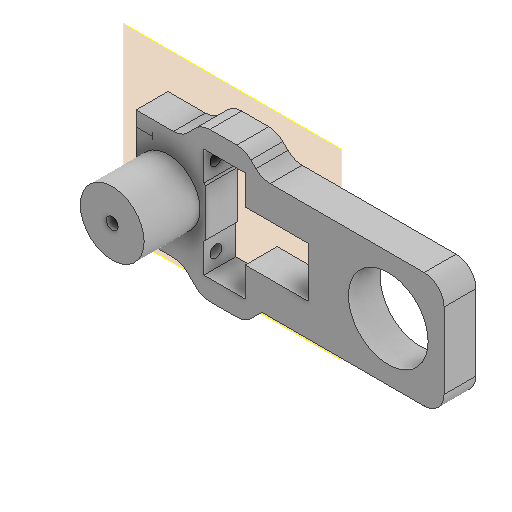
# Autodesk Inventor part: 30_Cube_Cube_Z_Focus_NEMA8_captive_objectivemount_v0
Saved by Autodesk Inventor 2022 (Build 260153000, 153)
## iProperties
Created: 2021-12-20
Part Number: 30_Cube_Cube_Z_Focus_NEMA8_captive_objectivemount_v0
Material: Generisch
Document SubType Name: Modeling
Designer: diederichbenedict
Density: 1 g/cm^3
Appearance: Vorgabe
Author: diederichbenedict
Autodesk Inventor part; units mm, degrees
ref_plane "YZ Plane" through (0, 0, 0) normal (1, 0, 0) x (0, 1, 0)
ref_plane "XZ Plane" through (0, 0, 0) normal (0, 1, 0) x (-1, 0, 0)
ref_plane "XY Plane" through (0, 0, 0) normal (0, 0, 1) x (1, 0, 0)
ref_plane "Arbeitsebene1" through (0, 0, 0) normal (0, 0, 1) x (1, 0, 0)
sketch "Skizze1" plane through (0, 0, 0) normal (0, 0, 1) x (1, 0, 0)
  arc A0 (9.5966, 13.5152) -> (9.0972, 14.0928) centre (8.4862, 13.06) ccw construction
  arc A1 (8.9755, 14.2862) -> (9.0972, 14.0928) centre (9.2245, 14.308) ccw construction
  line L0 (8.9755, 14.2862) -> (8.9453, 14.6318) construction
  arc A2 (8.9453, 14.6318) -> (8.6962, 14.86) centre (8.6962, 14.61) ccw construction
  line L1 (8.6962, 14.86) -> (8.2438, 14.86) construction
  arc A3 (8.2438, 14.86) -> (7.9947, 14.6318) centre (8.2438, 14.61) ccw construction
  line L2 (7.9947, 14.6318) -> (7.9627, 14.2652) construction
  arc A4 (7.8468, 14.0755) -> (7.9627, 14.2652) centre (7.7136, 14.287) ccw construction
  arc A5 (7.8468, 14.0755) -> (7.3759, 13.5152) centre (8.4862, 13.06) ccw construction
  arc A6 (7.1446, 13.36) -> (7.3759, 13.5152) centre (7.1446, 13.61) ccw construction
  line L3 (7.1446, 13.36) -> (6.47, 13.36) construction
  line L4 (6.47, 13.36) -> (5.97, 13.86) construction
  line L5 (5.97, 13.86) -> (5.97, 24.86) construction
  line L6 (5.97, 24.86) -> (6.47, 25.36) construction
  line L7 (6.47, 25.36) -> (7.1446, 25.36) construction
  arc A7 (7.3759, 25.2048) -> (7.1446, 25.36) centre (7.1446, 25.11) ccw construction
  arc A8 (7.3759, 25.2048) -> (7.8468, 24.6445) centre (8.4862, 25.66) ccw construction
  arc A9 (7.9627, 24.4548) -> (7.8468, 24.6445) centre (7.7136, 24.433) ccw construction
  line L8 (7.9627, 24.4548) -> (7.9947, 24.0882) construction
  arc A10 (7.9947, 24.0882) -> (8.2438, 23.86) centre (8.2438, 24.11) ccw construction
  line L9 (8.2438, 23.86) -> (8.6962, 23.86) construction
  arc A11 (8.6962, 23.86) -> (8.9453, 24.0882) centre (8.6962, 24.11) ccw construction
  line L10 (8.9453, 24.0882) -> (8.9755, 24.4338) construction
  arc A12 (9.0972, 24.6272) -> (8.9755, 24.4338) centre (9.2245, 24.412) ccw construction
  arc A13 (9.0972, 24.6272) -> (9.5966, 25.2048) centre (8.4862, 25.66) ccw construction
  arc A14 (9.8279, 25.36) -> (9.5966, 25.2048) centre (9.8279, 25.11) ccw construction
  line L11 (9.8279, 25.36) -> (10.97, 25.36) construction
  line L12 (10.97, 25.36) -> (10.97, 32.26) construction
  line L13 (10.97, 32.26) -> (10.37, 32.86) construction
  line L14 (10.37, 32.86) -> (6.97, 32.86) construction
  arc A15 (6.17, 32.86) -> (6.97, 32.86) centre (6.57, 33.16) ccw construction
  line L15 (6.17, 32.86) -> (1.57, 32.86) construction
  line L16 (1.57, 32.86) -> (0.97, 32.26) construction
  line L17 (0.97, 32.26) -> (0.97, 25.76) construction
  line L18 (0.97, 25.76) -> (1.37, 25.36) construction
  line L19 (1.37, 25.36) -> (1.37, 13.36) construction
  line L20 (1.37, 13.36) -> (0.97, 12.96) construction
  line L21 (0.97, 12.96) -> (0.97, 6.46) construction
  line L22 (0.97, 6.46) -> (1.57, 5.86) construction
  line L23 (1.57, 5.86) -> (10.37, 5.86) construction
  line L24 (10.37, 5.86) -> (10.97, 6.46) construction
  line L25 (10.97, 6.46) -> (10.97, 13.36) construction
  line L26 (10.97, 13.36) -> (9.8279, 13.36) construction
  arc A16 (9.5966, 13.5152) -> (9.8279, 13.36) centre (9.8279, 13.61) ccw construction
  line L27 (10.4528, 5.66) -> (1.4872, 5.66) construction
  line L28 (1.4872, 5.66) -> (0.77, 6.3772) construction
  line L29 (0.77, 6.3772) -> (0.77, 13.0428) construction
  line L30 (0.77, 13.0428) -> (1.17, 13.4428) construction
  line L31 (1.17, 13.4428) -> (1.17, 25.2772) construction
  line L32 (1.17, 25.2772) -> (0.77, 25.6772) construction
  line L33 (0.77, 25.6772) -> (0.77, 32.3428) construction
  line L34 (0.77, 32.3428) -> (1.4872, 33.06) construction
  line L35 (1.4872, 33.06) -> (6.2872, 33.06) construction
  arc A17 (6.2872, 33.06) -> (6.8528, 33.06) centre (6.57, 33.16) ccw construction
  line L36 (6.8528, 33.06) -> (10.4528, 33.06) construction
  line L37 (10.4528, 33.06) -> (11.17, 32.3428) construction
  line L38 (11.17, 32.3428) -> (11.17, 25.16) construction
  line L39 (11.17, 25.16) -> (9.8279, 25.16) construction
  arc A18 (9.8279, 25.16) -> (9.7816, 25.129) centre (9.8279, 25.11) ccw construction
  arc A19 (9.1991, 24.4551) -> (9.7816, 25.129) centre (8.4862, 25.66) ccw construction
  arc A20 (9.1991, 24.4551) -> (9.1747, 24.4164) centre (9.2245, 24.412) ccw construction
  line L40 (9.1747, 24.4164) -> (9.1445, 24.0708) construction
  arc A21 (8.6962, 23.66) -> (9.1445, 24.0708) centre (8.6962, 24.11) ccw construction
  line L41 (8.6962, 23.66) -> (8.2438, 23.66) construction
  arc A22 (7.7955, 24.0708) -> (8.2438, 23.66) centre (8.2438, 24.11) ccw construction
  line L42 (7.7955, 24.0708) -> (7.7634, 24.4373) construction
  arc A23 (7.7634, 24.4373) -> (7.7403, 24.4753) centre (7.7136, 24.433) ccw construction
  arc A24 (7.1909, 25.129) -> (7.7403, 24.4753) centre (8.4862, 25.66) ccw construction
  arc A25 (7.1909, 25.129) -> (7.1446, 25.16) centre (7.1446, 25.11) ccw construction
  line L43 (7.1446, 25.16) -> (6.5528, 25.16) construction
  line L44 (6.5528, 25.16) -> (6.17, 24.7772) construction
  line L45 (6.17, 24.7772) -> (6.17, 13.9428) construction
  line L46 (6.17, 13.9428) -> (6.5528, 13.56) construction
  line L47 (6.5528, 13.56) -> (7.1446, 13.56) construction
  arc A26 (7.1446, 13.56) -> (7.1909, 13.591) centre (7.1446, 13.61) ccw construction
  arc A27 (7.7403, 14.2447) -> (7.1909, 13.591) centre (8.4862, 13.06) ccw construction
  arc A28 (7.7403, 14.2447) -> (7.7634, 14.2827) centre (7.7136, 14.287) ccw construction
  line L48 (7.7634, 14.2827) -> (7.7955, 14.6492) construction
  arc A29 (8.2438, 15.06) -> (7.7955, 14.6492) centre (8.2438, 14.61) ccw construction
  line L49 (8.2438, 15.06) -> (8.6962, 15.06) construction
  arc A30 (9.1445, 14.6492) -> (8.6962, 15.06) centre (8.6962, 14.61) ccw construction
  line L50 (9.1445, 14.6492) -> (9.1747, 14.3036) construction
  arc A31 (9.1747, 14.3036) -> (9.1991, 14.2649) centre (9.2245, 14.308) ccw construction
  arc A32 (9.7816, 13.591) -> (9.1991, 14.2649) centre (8.4862, 13.06) ccw construction
  arc A33 (9.7816, 13.591) -> (9.8279, 13.56) centre (9.8279, 13.61) ccw construction
  line L51 (9.8279, 13.56) -> (11.17, 13.56) construction
  line L52 (11.17, 13.56) -> (11.17, 6.3772) construction
  line L53 (11.17, 6.3772) -> (10.4528, 5.66) construction
  line L54 (11.17, 25.66) -> (33.0091, 25.66)
  line L55 (11.17, 25.66) -> (33.0091, 25.66) construction
  line L56 (33.0091, 33.86) -> (15.3197, 33.86)
  line L57 (15.3197, 33.86) -> (11.1197, 38.06)
  line L58 (11.1197, 38.06) -> (0.1946, 38.06)
  line L59 (-16.23, 33.06) -> (-16.23, 19.36)
  line L60 (-16.23, 19.36) -> (1.17, 19.36)
  line L61 (1.17, 19.36) -> (1.17, 25.2772)
  line L62 (1.17, 25.2772) -> (0.77, 25.6772)
  line L63 (0.77, 25.6772) -> (0.77, 33.06)
  line L64 (0.77, 33.06) -> (11.17, 33.06)
  line L65 (11.17, 33.06) -> (11.17, 25.66)
  line L66 (36.7731, 34.36) -> (36.7731, 25.3561) projected
  line L67 (36.7731, 13.415) -> (36.7731, 4.36) projected
  line L68 (0.1946, 38.06) -> (-4.8054, 33.06)
  line L69 (0.1946, 38.06) -> (7.2656, 38.06) construction
  line L70 (-4.8054, 33.06) -> (-16.23, 33.06)
  line L71 (33.0091, 33.86) -> (33.0091, 25.66)
  line L72 (33.0091, 33.86) -> (61.0424, 33.86)
  line L73 (61.0424, 33.86) -> (61.0424, 19.36)
  line L74 (61.0424, 19.36) -> (57.0424, 19.36)
  line L75 (37.0424, 19.36) -> (27.0424, 19.36)
  line L76 (27.0424, 19.36) -> (27.0424, 25.66)
  circle A34 centre (47.0424, 19.36) radius 10
  point P0 (0, 0)
  point P1 (-2.0031, 19.36)
  point P2 (-4.8031, 19.36)
  dimension "d0" = 0.2
  dimension "d2" = 5
  dimension "d4" = 17
  dimension "d7" = 0.5
  dimension "d8" = 3.5
  dimension "d21" = 135
  dimension "d45" = 20
  dimension "d46" = 14
  dimension "d47" = 20
  dimension "d48" = 14.5
  constraints: 96 end point, 36 point on circle, 18 centre point, 7 point on line, 6 parallel, 4 perpendicular, 3 horizontal, 2 equal length, 1 collinear, 1 midpoint, 1 vertical, 43 other
  measures "d0" distance between parallel lines of L23 L27
  measures "d2" distance between parallel lines of L35 L58
  measures "d4" distance between parallel lines of L63 L59
  measures "d7" distance from line of L54 L38.end
  measures "d8" distance from line of L64.end L57
  measures "d21" angle of L68 L69
  measures "d45" diameter of A34
  measures "d46" distance from line of A34.centre L73
  measures "d47" distance from line of L76 A34.centre
  measures "d48" distance from line of L72 A34.centre
extrude "Extrusion1" add sketch "Skizze1" along normal blind 8 contours L65 L64 L63 L62 L61 L60 L59 L70 L68 L58 L57 L56 L71 L54 | L54 L71 L72 L73 L74 A34 L75 L76
sketch "Skizze2" plane through (-16.23, 19.36, 0) normal (-1, 0, 0) x (0, 0, 1)
  circle A0 centre (5, 10) radius 1.75 projected
  line L0 (0, 13.7) -> (0, 0) projected
  line L1 (0, 0) -> (8, 0) projected
  line L2 (8, 13.7) -> (8, 0) projected
  line L3 (0, 13.7) -> (8, 13.7) projected
  circle A1 centre (5, 10) radius 1.5
  point P0 (0, -19.36)
  dimension "d11" = 3
  constraints: 1 centre point
  measures "d11" diameter of A1
hole "Bohrung1" at (-16.23, 29.36, 5) direction (1, 0, 0) diameter 3 depth 20 tip angle 118 counterbore diameter 6 counterbore depth 4
mirror "Spiegeln2" about plane through (-16.23, 19.36, 0) normal (0, -1, 0) of "Extrusion1", "Bohrung1"
sketch "Skizze6" plane through (0, 0, 8) normal (0, 0, 1) x (1, 0, 0)
  line L0 (-16.23, 33.06) -> (-16.23, 5.66) projected
  circle A0 centre (-8.2208, 19.4223) radius 1.9812 projected
  circle A1 centre (-8.2208, 19.4223) radius 8.0094
  point P0 (0, 0)
  point P1 (-16.23, 19.36)
  constraints: 1 coincident, 1 midpoint, 3 other
extrude "Extrusion5" add sketch "Skizze6" along normal blind 14 contours A0 | A1
sketch "Skizze7" plane through (0, 0, 0) normal (0, 0, -1) x (-1, 0, 0)
  circle A0 centre (8.2208, 19.4223) radius 6
  circle A1 centre (8.2208, 19.4223) radius 1.9812 projected
  point P0 (0, 0)
  dimension "d34" = 12
  constraints: 1 centre point, 1 coincident
  measures "d34" diameter of A0
extrude "Extrusion6" cut sketch "Skizze7" against normal blind 20 contours A0 | A1
sketch "Skizze8" plane through (-7.7141, 19.36, 22) normal (0, 0, 1) x (1, 0, 0)
  circle A0 centre (-0.5067, 0.0623) radius 1.5
  circle A1 centre (-0.5067, 0.0623) radius 1.4224 projected
  point P0 (7.7141, -19.36)
  dimension "d37" = 3
  constraints: 1 centre point, 1 coincident
  measures "d37" diameter of A0
extrude "Extrusion7" cut sketch "Skizze8" against normal blind 15 contours A0 | A1
fillet "Rundung1" radius 5 9 edges at (61.0424, 33.86, 4) (61.0424, 4.86, 4) (11.1197, 0.66, 4) (0.1946, 0.66, 4) (-4.8054, 5.66, 4) (15.3197, 33.86, 4) (11.1197, 38.06, 4) (0.1946, 38.06, 4) (-4.8054, 33.06, 4)
